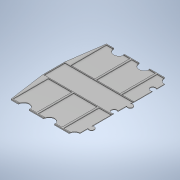
# Autodesk Inventor part: TI4_AgendaHolder
Saved by Autodesk Inventor 2021 (Build 250183000, 183)
## iProperties
Created: 2023-03-17
Part Number: TI4_AgendaHolder
Material: ABS Plastic
Document SubType Name: Modeling
Designer: Bradley
Density: 1.06 g/cm^3
Appearance: Smooth - Medium Gray
Author: Bradley
Autodesk Inventor part; units mm, degrees
ref_plane "YZ Plane" through (0, 0, 0) normal (1, 0, 0) x (0, 1, 0)
ref_plane "XZ Plane" through (0, 0, 0) normal (0, 1, 0) x (-1, 0, 0)
ref_plane "XY Plane" through (0, 0, 0) normal (0, 0, 1) x (1, 0, 0)
sketch "Sketch1" plane through (0, 0, 0) normal (0, 1, 0) x (-1, 0, 0)
  line L0 (126, 19.5) -> (-126, 19.5)
  line L1 (-126, 19.5) -> (-126, -19.5)
  line L2 (-126, -19.5) -> (126, -19.5)
  line L3 (126, -19.5) -> (126, 19.5)
  line L4 (126, 19.5) -> (-126, -19.5) construction
  line L5 (-126, 19.5) -> (126, -19.5) construction
  line L6 (127.6, -21.1) -> (-127.6, -21.1)
  line L7 (-127.6, -21.1) -> (-127.6, 21.1)
  line L8 (-127.6, 21.1) -> (127.6, 21.1)
  line L9 (127.6, 21.1) -> (127.6, -21.1)
  line L10 (-118, -88.7) -> (118, -88.7)
  line L11 (72.4, -21.1) -> (116.4, -21.1)
  line L12 (116.4, -21.1) -> (116.4, -87.1)
  line L13 (116.4, -87.1) -> (72.4, -87.1)
  line L14 (72.4, -87.1) -> (72.4, -21.1)
  line L15 (115.4, -86.1) -> (73.4, -86.1) construction
  line L16 (73.4, -86.1) -> (73.4, -22.1) construction
  line L17 (73.4, -22.1) -> (115.4, -22.1) construction
  line L18 (115.4, -22.1) -> (115.4, -86.1) construction
  line L19 (69.2, -87.1) -> (25.2, -87.1)
  line L20 (69.2, -21.1) -> (69.2, -87.1)
  line L21 (25.2, -87.1) -> (25.2, -21.1)
  line L22 (22, -87.1) -> (-22, -87.1)
  line L23 (22, -21.1) -> (22, -87.1)
  line L24 (-22, -87.1) -> (-22, -21.1)
  line L25 (-25.2, -87.1) -> (-69.2, -87.1)
  line L26 (-25.2, -21.1) -> (-25.2, -87.1)
  line L27 (-69.2, -87.1) -> (-69.2, -21.1)
  line L28 (-72.4, -87.1) -> (-116.4, -87.1)
  line L29 (-72.4, -21.1) -> (-72.4, -87.1)
  line L30 (-116.4, -87.1) -> (-116.4, -21.1)
  line L31 (127.6, -21.1) -> (118, -88.7)
  line L32 (-118, -88.7) -> (-127.6, -21.1)
  arc A0 (104.4, -88.7) -> (84.4, -88.7) centre (94.4, -88.7) ccw
  arc A1 (57.2, -88.7) -> (37.2, -88.7) centre (47.2, -88.7) ccw
  arc A2 (10, -88.7) -> (-10, -88.7) centre (0, -88.7) ccw
  arc A3 (-37.2, -88.7) -> (-57.2, -88.7) centre (-47.2, -88.7) ccw
  arc A4 (-84.4, -88.7) -> (-104.4, -88.7) centre (-94.4, -88.7) ccw
  point P0 (0, 0)
  point P1 (94.4, -86.1)
  point P2 (94.4, -87.1)
  point P3 (115.4, -54.1)
  point P4 (116.4, -54.1)
  point P5 (47.2, -87.1)
  point P6 (69.2, -54.1)
  point P7 (0, -87.1)
  point P8 (22, -54.1)
  point P9 (-47.2, -87.1)
  point P10 (-25.2, -54.1)
  point P11 (-94.4, -87.1)
  point P12 (-72.4, -54.1)
  point P13 (0, -87.1)
  point P14 (0, 0)
  point P15 (47.2, -87.1)
  point P16 (-47.2, -87.1)
  point P17 (-94.4, -87.1)
  point P18 (-104.2712, -87.1)
  point P19 (-116.4, -21.1)
  point P20 (-84.5288, -87.1)
  point P21 (-57.0712, -87.1)
  point P22 (-69.2, -21.1)
  point P23 (-37.3288, -87.1)
  point P24 (-9.8712, -87.1)
  point P25 (-22, -21.1)
  point P26 (9.8712, -87.1)
  point P27 (37.3288, -87.1)
  point P28 (25.2, -21.1)
  point P29 (57.0712, -87.1)
  point P30 (84.5288, -87.1)
  point P31 (104.2712, -87.1)
  dimension "d0" = 252
  dimension "d1" = 39
  dimension "d2" = 1.6
  dimension "d3" = 1.6
  dimension "d5" = 42
  dimension "d6" = 64
  dimension "d7" = 1
  dimension "d10" = 47.2
  dimension "d15" = 1
  dimension "d16" = 3.2
  dimension "d17" = 1.6
  dimension "d18" = 1.6
  dimension "d19" = 10
  constraints: 64 end point, 25 horizontal alignment, 16 parallel, 11 midpoint, 10 point on circle, 6 vertical alignment, 5 centre point, 4 collinear, 4 equal radius, 4 perpendicular, 3 horizontal, 1 coincident, 1 point on line, 22 other
  measures "d0" distance of L1.end L2.end
  measures "d1" distance of L0.end L1.end
  measures "d2" distance between parallel lines of L2 L6
  measures "d5" distance of L16.end L17.end
  measures "d6" distance of L15.end L16.end
  measures "d7" distance between parallel lines of L6 L17
  measures "d10" distance of L12.end L19.start
  measures "d15" distance between parallel lines of L12 L18
  measures "d16" distance between parallel lines of L20 L14
  measures "d17" distance from line of L12 L31.end
  measures "d18" distance from line of L32.start L30
  measures "d19" radius of A0
extrude "Extrusion1" add sketch "Sketch1" against normal blind 1 contours L3 L2 L1 L0 | L6 L7 L8 L9
extrude "Extrusion2" add sketch "Sketch1" along normal blind 1 contours L6 L7 L8 L9
extrude "Extrusion3" add sketch "Sketch1" against normal up to surface (1 mm away) contours L31 L10 A0 L13 L12 L6 | L12 L13 A0 L14 L6 | L14 L13 A0 L10 A1 L19 L20 L6 | L20 L19 A1 L21 L6 | L6 L30 L28 A4 L10 L32 | L21 L19 A1 L10 A2 L22 L23 L6 | L6 L29 L28 A4 L30 | L23 L22 A2 L24 L6 | L6 L27 L25 A3 L10 A4 L28 L29 | L24 L22 A2 L10 A3 L25 L26 L6 | L6 L26 L25 A3 L27
extrude "Extrusion4" add sketch "Sketch1" along normal up to surface (1 mm away) contours L31 L10 A0 L13 L12 L6 | L14 L13 A0 L10 A1 L19 L20 L6 | L6 L30 L28 A4 L10 L32 | L21 L19 A1 L10 A2 L22 L23 L6 | L6 L27 L25 A3 L10 A4 L28 L29 | L24 L22 A2 L10 A3 L25 L26 L6
pattern_circular "Circular Pattern1" count 2 over 360 about axis through (0, -10, 0) along (0, 1, 0) of "Extrusion3", "Extrusion4"
sketch "Sketch2" plane through (0, 0, 0) normal (0, 1, 0) x (-1, 0, 0)
  arc A0 (9.8712, -87.1) -> (-9.8712, -87.1) centre (0, -88.7) ccw projected
  arc A1 (-9.8712, 87.1) -> (9.8712, 87.1) centre (0, 88.7) ccw projected
  line L0 (116.4, 21.1) -> (72.4, 21.1) projected
  line L1 (72.4, 87.1) -> (72.4, 21.1) projected
  line L2 (84.5288, 87.1) -> (72.4, 87.1) projected
  arc A2 (84.4, 88.7) -> (84.5288, 87.1) centre (94.4, 88.7) ccw projected
  line L3 (57.2, 88.7) -> (84.4, 88.7) projected
  arc A3 (57.0712, 87.1) -> (57.2, 88.7) centre (47.2, 88.7) ccw projected
  line L4 (69.2, 87.1) -> (57.0712, 87.1) projected
  line L5 (69.2, 21.1) -> (69.2, 87.1) projected
  line L6 (69.2, 21.1) -> (25.2, 21.1) projected
  line L7 (25.2, 87.1) -> (25.2, 21.1) projected
  line L8 (37.3288, 87.1) -> (25.2, 87.1) projected
  arc A4 (37.2, 88.7) -> (37.3288, 87.1) centre (47.2, 88.7) ccw projected
  line L9 (10, 88.7) -> (37.2, 88.7) projected
  arc A5 (9.8712, 87.1) -> (10, 88.7) centre (0, 88.7) ccw projected
  line L10 (22, 87.1) -> (9.8712, 87.1) projected
  line L11 (22, 21.1) -> (22, 87.1) projected
  line L12 (22, 21.1) -> (-22, 21.1) projected
  line L13 (-22, 87.1) -> (-22, 21.1) projected
  line L14 (-9.8712, 87.1) -> (-22, 87.1) projected
  arc A6 (-10, 88.7) -> (-9.8712, 87.1) centre (0, 88.7) ccw projected
  line L15 (-37.2, 88.7) -> (-10, 88.7) projected
  arc A7 (-37.3288, 87.1) -> (-37.2, 88.7) centre (-47.2, 88.7) ccw projected
  line L16 (-25.2, 87.1) -> (-37.3288, 87.1) projected
  line L17 (-25.2, 21.1) -> (-25.2, 87.1) projected
  line L18 (-25.2, 21.1) -> (-69.2, 21.1) projected
  line L19 (-69.2, 87.1) -> (-69.2, 21.1) projected
  line L20 (-57.0712, 87.1) -> (-69.2, 87.1) projected
  arc A8 (-57.2, 88.7) -> (-57.0712, 87.1) centre (-47.2, 88.7) ccw projected
  line L21 (-84.4, 88.7) -> (-57.2, 88.7) projected
  arc A9 (-84.5288, 87.1) -> (-84.4, 88.7) centre (-94.4, 88.7) ccw projected
  line L22 (-72.4, 87.1) -> (-84.5288, 87.1) projected
  line L23 (-72.4, 21.1) -> (-72.4, 87.1) projected
  line L24 (-72.4, 21.1) -> (-116.4, 21.1) projected
  line L25 (-116.4, 87.1) -> (-116.4, 21.1) projected
  line L26 (-104.2712, 87.1) -> (-116.4, 87.1) projected
  arc A10 (-104.4, 88.7) -> (-104.2712, 87.1) centre (-94.4, 88.7) ccw projected
  line L27 (-118, 88.7) -> (-104.4, 88.7) projected
  line L28 (-127.6, 21.1) -> (-118, 88.7) projected
  line L29 (-127.6, 21.1) -> (-127.6, -21.1) projected
  line L30 (-118, -88.7) -> (-127.6, -21.1) projected
  line L31 (-104.4, -88.7) -> (-118, -88.7) projected
  arc A11 (-104.2712, -87.1) -> (-104.4, -88.7) centre (-94.4, -88.7) ccw projected
  line L32 (-116.4, -87.1) -> (-104.2712, -87.1) projected
  line L33 (-116.4, -21.1) -> (-116.4, -87.1) projected
  line L34 (-116.4, -21.1) -> (-72.4, -21.1) projected
  line L35 (-72.4, -87.1) -> (-72.4, -21.1) projected
  line L36 (-84.5288, -87.1) -> (-72.4, -87.1) projected
  arc A12 (-84.4, -88.7) -> (-84.5288, -87.1) centre (-94.4, -88.7) ccw projected
  line L37 (-57.2, -88.7) -> (-84.4, -88.7) projected
  arc A13 (-57.0712, -87.1) -> (-57.2, -88.7) centre (-47.2, -88.7) ccw projected
  line L38 (-69.2, -87.1) -> (-57.0712, -87.1) projected
  line L39 (-69.2, -21.1) -> (-69.2, -87.1) projected
  line L40 (-69.2, -21.1) -> (-25.2, -21.1) projected
  line L41 (-25.2, -87.1) -> (-25.2, -21.1) projected
  line L42 (-37.3288, -87.1) -> (-25.2, -87.1) projected
  arc A14 (-37.2, -88.7) -> (-37.3288, -87.1) centre (-47.2, -88.7) ccw projected
  line L43 (-10, -88.7) -> (-37.2, -88.7) projected
  arc A15 (-9.8712, -87.1) -> (-10, -88.7) centre (0, -88.7) ccw projected
  line L44 (-22, -87.1) -> (-9.8712, -87.1) projected
  line L45 (-22, -21.1) -> (-22, -87.1) projected
  line L46 (-22, -21.1) -> (22, -21.1) projected
  line L47 (22, -87.1) -> (22, -21.1) projected
  line L48 (9.8712, -87.1) -> (22, -87.1) projected
  arc A16 (10, -88.7) -> (9.8712, -87.1) centre (0, -88.7) ccw projected
  line L49 (37.2, -88.7) -> (10, -88.7) projected
  arc A17 (37.3288, -87.1) -> (37.2, -88.7) centre (47.2, -88.7) ccw projected
  line L50 (25.2, -87.1) -> (37.3288, -87.1) projected
  line L51 (25.2, -21.1) -> (25.2, -87.1) projected
  line L52 (25.2, -21.1) -> (69.2, -21.1) projected
  line L53 (69.2, -87.1) -> (69.2, -21.1) projected
  line L54 (57.0712, -87.1) -> (69.2, -87.1) projected
  arc A18 (57.2, -88.7) -> (57.0712, -87.1) centre (47.2, -88.7) ccw projected
  line L55 (84.4, -88.7) -> (57.2, -88.7) projected
  arc A19 (84.5288, -87.1) -> (84.4, -88.7) centre (94.4, -88.7) ccw projected
  line L56 (72.4, -87.1) -> (84.5288, -87.1) projected
  line L57 (72.4, -21.1) -> (72.4, -87.1) projected
  line L58 (72.4, -21.1) -> (116.4, -21.1) projected
  line L59 (116.4, -87.1) -> (116.4, -21.1) projected
  line L60 (104.2712, -87.1) -> (116.4, -87.1) projected
  arc A20 (104.4, -88.7) -> (104.2712, -87.1) centre (94.4, -88.7) ccw projected
  line L61 (118, -88.7) -> (104.4, -88.7) projected
  line L62 (127.6, -21.1) -> (118, -88.7) projected
  line L63 (127.6, -21.1) -> (127.6, 21.1) projected
  line L64 (118, 88.7) -> (127.6, 21.1) projected
  line L65 (104.4, 88.7) -> (118, 88.7) projected
  arc A21 (104.2712, 87.1) -> (104.4, 88.7) centre (94.4, 88.7) ccw projected
  line L66 (116.4, 87.1) -> (104.2712, 87.1) projected
  line L67 (116.4, 21.1) -> (116.4, 87.1) projected
  line L68 (126, 19.5) -> (126, -19.5) projected
  line L69 (126, -19.5) -> (-126, -19.5) projected
  line L70 (-126, -19.5) -> (-126, 19.5) projected
  line L71 (-126, 19.5) -> (126, 19.5) projected
  arc A22 (0, -64) -> (0, -56) centre (3, -60) ccw
  arc A23 (0, -8.3173) -> (0, -15.6827) centre (-3, -12) ccw
  arc A24 (0, 8) -> (0, 16) centre (3, 12) ccw
  arc A25 (0, 63.6827) -> (0, 56.3173) centre (-3, 60) ccw
  line L72 (0, 78.7) -> (0, 63.6827)
  line L73 (0, 56.3173) -> (0, 16)
  line L74 (22, 21.1) -> (-22, 21.1) projected
  line L75 (0, 8) -> (0, -8.3173)
  line L76 (0, -15.6827) -> (0, -56)
  line L77 (0, -64) -> (0, -78.7)
  arc A26 (-37.3288, -87.1) -> (-57.0712, -87.1) centre (-47.2, -88.7) ccw projected
  arc A27 (-84.5288, -87.1) -> (-104.2712, -87.1) centre (-94.4, -88.7) ccw projected
  line L78 (-116.4, 87.1) -> (-116.4, 21.1) projected
  line L79 (-72.4, 21.1) -> (-116.4, 21.1) projected
  line L80 (-72.4, 21.1) -> (-72.4, 87.1) projected
  line L81 (-72.4, 87.1) -> (-84.5288, 87.1) projected
  arc A28 (-104.2712, 87.1) -> (-84.5288, 87.1) centre (-94.4, 88.7) ccw projected
  line L82 (-104.2712, 87.1) -> (-116.4, 87.1) projected
  line L83 (-25.2, 87.1) -> (-37.3288, 87.1) projected
  arc A29 (-57.0712, 87.1) -> (-37.3288, 87.1) centre (-47.2, 88.7) ccw projected
  line L84 (-57.0712, 87.1) -> (-69.2, 87.1) projected
  line L85 (-69.2, 87.1) -> (-69.2, 21.1) projected
  line L86 (-25.2, 21.1) -> (-69.2, 21.1) projected
  line L87 (-25.2, 21.1) -> (-25.2, 87.1) projected
  point P0 (0, 0)
  point P1 (-9.8712, -87.1)
  dimension "d31" = 12
  dimension "d32" = 12
  dimension "d33" = 5
  dimension "d34" = 4.75
  dimension "d35" = 3
  dimension "d36" = 3
  dimension "d41" = 60
  dimension "d42" = 60
  dimension "d43" = 5
  dimension "d44" = 4.75
  constraints: 10 end point, 10 point on circle, 5 collinear, 4 centre point, 2 equal radius, 2 vertical alignment, 1 perpendicular, 1 point on line, 1 vertical
  measures "d31" vertical distance of A23.centre point (0, 0)
  measures "d32" vertical distance of A24.centre point (0, 0)
  measures "d33" radius of A24
  measures "d34" radius of A23
  measures "d35" horizontal distance of A24.centre point (0, 0)
  measures "d36" distance from line of A23.centre L75
  measures "d41" vertical distance of A22.centre point (0, 0)
  measures "d42" vertical distance of A25.centre point (0, 0)
  measures "d43" radius of A22
  measures "d44" radius of A25
extrude "Extrusion5" cut sketch "Sketch2" along normal through all both and the other way through all contours A0 L44 L45 L46 L76 A22 L77 | A15 L43 A14 L42 L41 L40 L39 L38 A13 L37 A12 L36 L35 L34 L33 L32 A11 L31 L30 L29 L28 L27 A10 L26 L25 L24 L23 L22 A9 L21 A8 L20 L19 L18 L17 L16 A7 L15 A6 L14 L13 L12 L73 L71 L70 L69 L76 L46 L45 L44 | L69 L70 L71 L73 A24 L75 A23 L76 | A26 L38 L39 L40 L41 L42 | L12 L13 L14 A1 L72 A25 L73 | A27 L32 L33 L34 L35 L36 | L16 L17 L18 L19 L20 A29 | A28 L22 L23 L24 L25 L26
equation "\"d3\" = d2"
equation "\"d16\" = 2 * d3"
equation "\"d17\" = d2"
equation "\"d18\" = d2"
equation "\"d32\" = d31"
equation "\"d36\" = d35"
equation "\"d42\" = d41"
body "Solid1"
